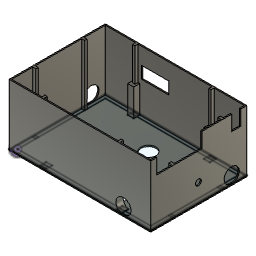
matek_enclosure (Autodesk Fusion 360 design; units mm, degrees)
Autodesk Fusion 360 part; units mm, degrees
sketch "Sketch1" plane through (0, 0, 0) normal (0, 0, 1) x (1, 0, 0)
  line L0 (0, 0) -> (44, 0)
  line L1 (44, 0) -> (44, 29)
  line L2 (44, 29) -> (0, 29)
  line L3 (0, 29) -> (0, 0)
  line L4 (45, -1) -> (45, 30)
  line L5 (45, 30) -> (-1, 30)
  line L6 (-1, 30) -> (-1, -1)
  line L7 (-1, -1) -> (45, -1)
  line L8 (45.4, -1.4) -> (45.4, 30.4)
  line L9 (45.4, 30.4) -> (-1.4, 30.4)
  line L10 (-1.4, 30.4) -> (-1.4, -1.4)
  line L11 (-1.4, -1.4) -> (45.4, -1.4)
  line L12 (9, 30) -> (9, 29)
  line L13 (-1, 23) -> (0, 23)
  line L14 (9.8, 30) -> (9.8, 29)
  line L15 (-1, 22.2) -> (0, 22.2)
  line L16 (34.2, 30) -> (34.2, 29)
  line L17 (35, 30) -> (35, 29)
  line L18 (44, 23) -> (45, 23)
  line L19 (44, 22.2) -> (45, 22.2)
  line L20 (44, 6.8) -> (45, 6.8)
  line L21 (44, 6) -> (45, 6)
  line L22 (35, 0) -> (35, -1)
  line L23 (34.2, 0) -> (34.2, -1)
  line L24 (9, 0) -> (9, -1)
  line L25 (9.8, 0) -> (9.8, -1)
  line L26 (-1, 6.8) -> (0, 6.8)
  line L27 (-1, 6) -> (0, 6)
  line L28 (33.6, 30) -> (35.6, 30)
  line L29 (35.6, 30) -> (35.6, 28)
  line L30 (35.6, 28) -> (33.6, 28)
  line L31 (33.6, 28) -> (33.6, 30)
  line L32 (8.4, 30) -> (10.4, 30)
  line L33 (10.4, 30) -> (10.4, 28)
  line L34 (10.4, 28) -> (8.4, 28)
  line L35 (8.4, 28) -> (8.4, 30)
  line L36 (33.6, -1) -> (35.6, -1)
  line L37 (35.6, -1) -> (35.6, 1)
  line L38 (35.6, 1) -> (33.6, 1)
  line L39 (33.6, 1) -> (33.6, -1)
  line L40 (8.4, -1) -> (10.4, -1)
  line L41 (10.4, -1) -> (10.4, 1)
  line L42 (10.4, 1) -> (8.4, 1)
  line L43 (8.4, 1) -> (8.4, -1)
  dimension "d1" = 29
  dimension "d2" = 44
  dimension "d3" = 1
  dimension "d4" = 1.4
  dimension "d5" = 9
  dimension "d6" = 0.8
  dimension "d7" = 9
  dimension "d8" = 0.8
  dimension "d9" = 6
  dimension "d10" = 0.8
  dimension "d11" = 6
  dimension "d12" = 0.8
  dimension "d13" = 9
  dimension "d14" = 0.8
  dimension "d15" = 6
  dimension "d16" = 0.8
  dimension "d17" = 6
  dimension "d18" = 0.8
  dimension "d19" = 9
  dimension "d20" = 0.8
  dimension "d64" = 2
  dimension "d65" = 2
  dimension "d66" = 0.6
  dimension "d67" = 2
  dimension "d68" = 2
  dimension "d69" = 0.6
  dimension "d70" = 2
  dimension "d71" = 2
  dimension "d72" = 0.6
  dimension "d73" = 2
  dimension "d74" = 2
  dimension "d75" = 0.6
  constraint horizontal L0
  constraint vertical L1
  constraint horizontal L2
  constraint vertical L3
  constraint coincident L0.start L3.end
  constraint coincident L5 L12.start
  constraint coincident L2 L12.end
  constraint perpendicular L2 L12
  constraint coincident L6 L13.start
  constraint coincident L3 L13.end
  constraint perpendicular L3 L13
  constraint coincident L5 L14.start
  constraint coincident L2 L14.end
  constraint perpendicular L2 L14
  constraint coincident L6 L15.start
  constraint coincident L3 L15.end
  constraint perpendicular L3 L15
  constraint coincident L5 L16.start
  constraint coincident L2 L16.end
  constraint perpendicular L2 L16
  constraint coincident L5 L17.start
  constraint coincident L2 L17.end
  constraint perpendicular L2 L17
  constraint coincident L1 L18.start
  constraint coincident L4 L18.end
  constraint perpendicular L4 L18
  constraint coincident L1 L19.start
  constraint coincident L4 L19.end
  constraint perpendicular L4 L19
  constraint coincident L1 L20.start
  constraint coincident L4 L20.end
  constraint perpendicular L4 L20
  constraint coincident L1 L21.start
  constraint coincident L4 L21.end
  constraint perpendicular L4 L21
  constraint coincident L0 L22.start
  constraint coincident L7 L22.end
  constraint perpendicular L7 L22
  constraint coincident L0 L23.start
  constraint coincident L7 L23.end
  constraint perpendicular L7 L23
  constraint coincident L0 L24.start
  constraint coincident L7 L24.end
  constraint perpendicular L7 L24
  constraint coincident L0 L25.start
  constraint coincident L7 L25.end
  constraint perpendicular L7 L25
  constraint coincident L6 L26.start
  constraint coincident L3 L26.end
  constraint perpendicular L3 L26
  constraint coincident L6 L27.start
  constraint coincident L3 L27.end
  constraint perpendicular L3 L27
  constraint horizontal L28
  constraint vertical L29
  constraint horizontal L30
  constraint vertical L31
  constraint coincident L5 L28.start
  constraint horizontal L32
  constraint vertical L33
  constraint horizontal L34
  constraint vertical L35
  constraint coincident L5 L32.start
  constraint horizontal L36
  constraint vertical L37
  constraint horizontal L38
  constraint vertical L39
  constraint coincident L7 L36.start
  constraint horizontal L40
  constraint vertical L41
  constraint horizontal L42
  constraint vertical L43
  constraint coincident L7 L40.start
  measures "d1" distance of L0.start L2.end
  measures "d2" distance of L1.end L2.end
  measures "d5" distance of L3 L12
  measures "d6" distance of L12 L14
  measures "d7" distance of L1 L17
  measures "d8" distance of L16 L17.start
  measures "d9" distance of L2 L18
  measures "d10" distance of L18 L19
  measures "d11" distance of L0 L21
  measures "d12" distance of L20 L21
  measures "d13" distance of L1 L22
  measures "d14" distance of L22 L23
  measures "d15" distance of L2 L13
  measures "d16" distance of L13 L15
  measures "d17" distance of L0 L27
  measures "d18" distance of L26 L27
  measures "d19" distance of L3 L24
  measures "d20" distance of L24 L25
  measures "d64" distance of L28.end L29.end
  measures "d65" distance of L29.end L30.end
  measures "d66" distance of L17 L29
  measures "d67" distance of L33.end L34.end
  measures "d68" distance of L32.end L33.end
  measures "d69" distance of L14 L33
  measures "d70" distance of L37.end L38.end
  measures "d71" distance of L36.start L38.end
  measures "d72" distance of L23 L39
  measures "d73" distance of L41.end L42.end
  measures "d74" distance of L40.end L41.end
  measures "d75" distance of L24 L43
extrude "Extrude1" add sketch "Sketch1" along normal blind 20
extrude "Extrude2" add sketch "Sketch1" against normal blind 0.4 contours L0 L41 L42 L43 | L0 L7 L24 L40 L43 | L0 L7 L24 L25 L40 | L0 L7 L25 L40 L41 | L0 L3 L6 L7 L27 L43 | L0 L1 L2 L3 L29 L30 L31 L33 L34 L35 L37 L38 L39 L41 L42 L43 | L0 L7 L39 L41 | L0 L37 L38 L39 | L0 L7 L23 L36 L39 | L3 L6 L26 L27 | L0 L7 L22 L23 L36 | L3 L6 L15 L26 | L0 L7 L22 L36 L37 | L3 L6 L13 L15 | L0 L1 L4 L7 L21 L37 | L2 L3 L5 L6 L13 L35 | L1 L4 L20 L21 | L2 L5 L12 L32 L35 | L2 L33 L34 L35 | L1 L4 L19 L20 | L2 L5 L12 L14 L32 | L1 L4 L18 L19 | L2 L5 L14 L32 L33 | L1 L2 L4 L5 L18 L29 | L2 L5 L31 L33 | L2 L5 L16 L28 L31 | L2 L29 L30 L31 | L2 L5 L17 L28 L29 | L2 L5 L16 L17 L28 | L8 L9 L10 L11
extrude "Extrude3" add sketch "Sketch1" along normal blind 20 contours L0 L7 L24 L25 L40 | L3 L6 L26 L27 | L0 L7 L22 L23 L36 | L3 L6 L13 L15 | L1 L4 L20 L21 | L2 L5 L12 L14 L32 | L1 L4 L18 L19 | L2 L5 L16 L17 L28
sketch "Sketch2" plane through (45.4, 0, 0) normal (1, 0, 0) x (0, 1, 0)
  line L0 (30.4, -0.4) -> (30.4, 20)
  line L1 (30.4, 20) -> (-1.4, 20)
  line L2 (-1.4, 20) -> (-1.4, -0.4)
  line L3 (-1.4, -0.4) -> (30.4, -0.4)
  line L4 (-1.4, 20) -> (30.4, 20)
  line L5 (30.4, 20) -> (30.4, 15)
  line L6 (30.4, 15) -> (-1.4, 15)
  line L7 (-1.4, 15) -> (-1.4, 20)
  line L8 (15.6, 20) -> (15.6, 15)
  line L9 (25.4, 20) -> (25.4, 15)
  line L10 (0.6, 20) -> (0.6, 15)
  line L11 (28.4, 20) -> (28.4, 15)
  dimension "d27" = 5
  dimension "d28" = 17
  dimension "d29" = 5
  dimension "d30" = 2
  dimension "d31" = 2
  constraint horizontal L4
  constraint vertical L5
  constraint horizontal L6
  constraint vertical L7
  constraint coincident L0 L5.end
  constraint coincident L1.end L2.start
  constraint coincident L4 L8.start
  constraint coincident L6 L8.end
  constraint perpendicular L6 L8
  constraint coincident L1 L9.start
  constraint coincident L6 L9.end
  constraint perpendicular L6 L9
  constraint coincident L4 L10.start
  constraint coincident L6 L10.end
  constraint perpendicular L6 L10
  constraint coincident L4 L11.start
  constraint coincident L6 L11.end
  constraint perpendicular L6 L11
  measures "d27" distance of L4 L6
  measures "d28" distance of L7 L8
  measures "d29" distance of L5 L9
  measures "d30" distance of L7 L10
  measures "d31" distance of L5 L11
extrude "Extrude4" cut sketch "Sketch2" against normal blind 3 contours L1 L4 L6 L9 L11 | L1 L4 L6 L8 L10
sketch "Sketch3" plane through (45.4, 0, 0) normal (1, 0, 0) x (0, 1, 0)
  line L0 (15.6, 20) -> (15.6, 15)
  line L1 (15.6, 15) -> (0.6, 15)
  line L2 (0.6, 15) -> (0.6, 20)
  line L3 (0.6, 20) -> (-1.4, 20)
  line L4 (-1.4, 20) -> (-1.4, -0.4)
  line L5 (-1.4, -0.4) -> (30.4, -0.4)
  line L6 (30.4, -0.4) -> (30.4, 20)
  line L7 (30.4, 20) -> (28.4, 20)
  line L8 (28.4, 20) -> (28.4, 15)
  line L9 (28.4, 15) -> (25.4, 15)
  line L10 (25.4, 15) -> (25.4, 20)
  line L11 (25.4, 20) -> (15.6, 20)
  circle A0 centre (25.4, 2.5) radius 2.5
  line L12 (-1.4, 0) -> (30.4, 0)
  dimension "d34" = 5
  dimension "d35" = 5
  constraint tangent A0 L12
  measures "d34" diameter of A0
  measures "d35" distance of L6 A0.centre
extrude "Extrude5" cut sketch "Sketch3" against normal blind 54 contours A0
sketch "Sketch4" plane through (0, -1.4, 0) normal (0, -1, 0) x (1, 0, 0)
  line L0 (45.4, -0.4) -> (45.4, 20)
  line L1 (45.4, 20) -> (-1.4, 20)
  line L2 (-1.4, 20) -> (-1.4, -0.4)
  line L3 (-1.4, -0.4) -> (45.4, -0.4)
  circle A0 centre (36.4, 2.5) radius 2.5
  line L4 (-1.4, 0) -> (45.4, 0)
  dimension "d38" = 5
  dimension "d39" = 9
  constraint tangent A0 L4
  measures "d38" diameter of A0
  measures "d39" distance of L0 A0.centre
sketch "Sketch5" plane through (0, 0, 0) normal (0, 0, 1) x (1, 0, 0)
  line L0 (44, 0) -> (41, 0)
  line L1 (41, 0) -> (41, 8)
  line L2 (41, 8) -> (44, 8)
  line L3 (44, 8) -> (44, 0)
  line L4 (32.5, 8) -> (26.5, 8)
  line L5 (26.5, 8) -> (26.5, 0)
  line L6 (26.5, 0) -> (32.5, 0)
  line L7 (32.5, 0) -> (32.5, 8)
  line L8 (44, 0) -> (44, 29)
  point P0 (44, 0)
  dimension "d42" = 3
  dimension "d43" = 8
  dimension "d44" = 11.5
  dimension "d45" = 8
  dimension "d46" = 6
  constraint horizontal L0
  constraint vertical L1
  constraint horizontal L2
  constraint vertical L3
  constraint coincident P0 L0.start
  constraint horizontal L4
  constraint vertical L5
  constraint horizontal L6
  constraint vertical L7
  constraint collinear L2 L4
  measures "d42" distance of P0 L1
  measures "d43" distance of L0.end L1.end
  measures "d44" distance of L7 L8
  measures "d45" distance of L4.end L5.end
  measures "d46" distance of L4.start L4.end
extrude "Extrude7" cut sketch "Sketch5" against normal blind 2
sketch "Sketch6" plane through (45.4, 0, 0) normal (1, 0, 0) x (0, 1, 0)
  circle A0 centre (25.4, 2.5) radius 2.5
  line L0 (15.6, 20) -> (15.6, 15)
  line L1 (15.6, 15) -> (0.6, 15)
  line L2 (0.6, 15) -> (0.6, 20)
  line L3 (0.6, 20) -> (-1.4, 20)
  line L4 (-1.4, 20) -> (-1.4, -0.4)
  line L5 (-1.4, -0.4) -> (30.4, -0.4)
  line L6 (30.4, -0.4) -> (30.4, 20)
  line L7 (30.4, 20) -> (28.4, 20)
  line L8 (28.4, 20) -> (28.4, 15)
  line L9 (28.4, 15) -> (25.4, 15)
  line L10 (25.4, 15) -> (25.4, 20)
  line L11 (25.4, 20) -> (15.6, 20)
  circle A1 centre (14.4, 6) radius 1
  line L12 (-1.4, 0) -> (30.4, 0)
  dimension "d49" = 2
  dimension "d50" = 6
  dimension "d51" = 16
  measures "d49" diameter of A1
  measures "d50" distance of A1.centre L12
  measures "d51" distance of L6 A1.centre
extrude "Extrude8" cut sketch "Sketch6" against normal blind 3 contours A1
sketch "Sketch7" plane through (0, 0, -0.4) normal (0, 0, -1) x (1, 0, 0)
  line L0 (44, 0) -> (44, -8)
  line L1 (44, -8) -> (41, -8)
  line L2 (41, -8) -> (41, 0)
  line L3 (41, 0) -> (44, 0)
  line L4 (32.5, -8) -> (26.5, -8)
  line L5 (26.5, -8) -> (26.5, 0)
  line L6 (26.5, 0) -> (32.5, 0)
  line L7 (32.5, 0) -> (32.5, -8)
  line L8 (45.4, 1.4) -> (-1.4, 1.4)
  line L9 (-1.4, 1.4) -> (-1.4, -30.4)
  line L10 (-1.4, -30.4) -> (45.4, -30.4)
  line L11 (45.4, -30.4) -> (45.4, 1.4)
  circle A0 centre (22.278, -21) radius 2.5
  line L12 (44, -29) -> (0, -29)
  dimension "d54" = 5
  dimension "d55" = 8
  measures "d54" diameter of A0
  measures "d55" distance of A0.centre L12
extrude "Extrude9" cut sketch "Sketch7" against normal blind 2 contours A0
sketch "Sketch8" plane through (0, 30.4, 0) normal (0, 1, 0) x (-1, 0, 0)
  line L0 (1.4, -0.4) -> (1.4, 20)
  line L1 (1.4, 20) -> (-45.4, 20)
  line L2 (-45.4, 20) -> (-45.4, -0.4)
  line L3 (-45.4, -0.4) -> (1.4, -0.4)
  line L4 (-11, 10.5) -> (-20, 10.5)
  line L5 (-20, 10.5) -> (-20, 14.5)
  line L6 (-20, 14.5) -> (-11, 14.5)
  line L7 (-11, 14.5) -> (-11, 10.5)
  line L8 (-45.4, 0) -> (1.4, 0)
  dimension "d58" = 11
  dimension "d59" = 20
  dimension "d60" = 4
  dimension "d61" = 10.5
  constraint horizontal L4
  constraint vertical L5
  constraint horizontal L6
  constraint vertical L7
  measures "d58" distance of L7 origin
  measures "d59" distance of origin L5
  measures "d60" distance of L4.end L5.end
  measures "d61" distance of L4 L8
extrude "Extrude10" cut sketch "Sketch8" against normal blind 2 contours L4 L5 L6 L7
sketch "Sketch9" plane through (0, 0, 0) normal (0, 0, 1) x (1, 0, 0)
extrude "Extrude11" add sketch "Sketch1" along normal blind 9 contours L0 L41 L42 L43 | L0 L7 L24 L40 L43 | L0 L7 L25 L40 L41 | L0 L37 L38 L39 | L0 L7 L23 L36 L39 | L0 L7 L22 L36 L37 | L2 L5 L12 L32 L35 | L2 L33 L34 L35 | L2 L5 L14 L32 L33 | L2 L5 L16 L28 L31 | L2 L29 L30 L31 | L2 L5 L17 L28 L29
extrude "Extrude6" cut sketch "Sketch4" against normal blind 6 contours A0
named bodies: "matek_enclosure"
